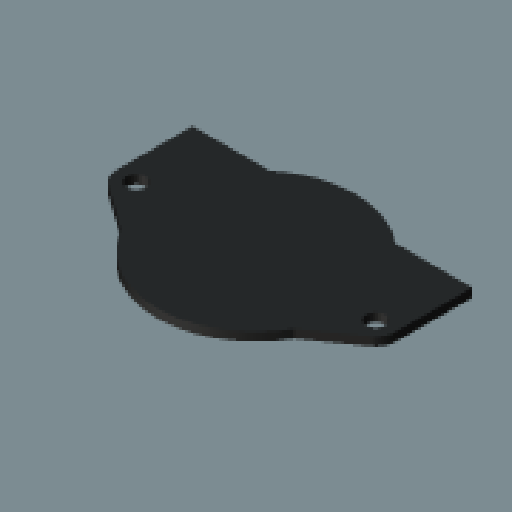
# Autodesk Inventor part: Mellow Fly SHT36
Saved by Autodesk Inventor 2023.2 (Build 272271000, 271)
## iProperties
Created: 2023-02-06
Part Number: Mellow Fly SHT36
Material: Copper, Alloy
Document SubType Name: Modeling
Designer: remop
Density: 8.92 g/cm^3
Appearance: Glossy - Black
Author: remop
Autodesk Inventor part; units mm, degrees
ref_plane "YZ Plane" through (0, 0, 0) normal (1, 0, 0) x (0, 1, 0)
ref_plane "XZ Plane" through (0, 0, 0) normal (0, 1, 0) x (-1, 0, 0)
ref_plane "XY Plane" through (0, 0, 0) normal (0, 0, 1) x (1, 0, 0)
sketch "Sketch1" plane through (0, 0, 0) normal (0, 1, 0) x (-1, 0, 0)
  circle A0 centre (-21.92, 0) radius 1.75
  circle A1 centre (21.92, 0) radius 1.75
  circle A2 centre (0, 0) radius 18.13
  circle A3 centre (-21.92, 0) radius 3.715
  circle A4 centre (21.92, 0) radius 3.715
  line L0 (-25.635, 0) -> (-25.635, -14)
  line L1 (-25.635, -14) -> (-11.5194, -14)
  line L2 (11.5194, -14) -> (25.635, -14)
  line L3 (25.635, -14) -> (25.635, 0)
  line L4 (24.0715, 3.0286) -> (15.7877, 8.9132)
  line L5 (-24.0715, 3.0286) -> (-15.7877, 8.9132)
  dimension "d0" = 3.5
  dimension "d1" = 43.84
  dimension "d2" = 21.92
  dimension "d3" = 36.26
  dimension "d4" = 51.27
  dimension "d5" = 14
  dimension "d7" = 35.389
  constraints: 12 end point, 8 point on circle, 5 centre point, 4 tangent, 3 coincident, 2 equal length, 2 horizontal alignment, 2 point on line, 1 equal radius, 1 perpendicular, 1 vertical
  measures "d0" diameter of A0
  measures "d1" distance of A1.centre A0.centre
  measures "d2" distance of point (0, 0) A1.centre
  measures "d3" diameter of A2
  measures "d4" distance between parallel lines of L3 L0
  measures "d5" distance from line of L1 point (0, 0)
  measures "d7" angle of L2 L4
extrude "Extrusion1" add sketch "Sketch1" along normal blind 1.6
equation "\"d2\" = 0.5 * d1"
body "Solid1"
